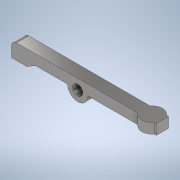
# Autodesk Inventor part: Peça8
Saved by Autodesk Inventor 2021 (Build 250183000, 183)
## iProperties
Created: 2021-07-18
Part Number: Peça8
Material: Liga de aço
Document SubType Name: Modeling
Designer: Giovanni
Density: 7.73 g/cm^3
Appearance: Galvanizado
Author: Giovanni
Autodesk Inventor part; units mm, degrees
ref_plane "YZ Plane" through (0, 0, 0) normal (1, 0, 0) x (0, 1, 0)
ref_plane "XZ Plane" through (0, 0, 0) normal (0, 1, 0) x (-1, 0, 0)
ref_plane "XY Plane" through (0, 0, 0) normal (0, 0, 1) x (1, 0, 0)
sketch "Esboço1" plane through (0, 0, 0) normal (0, 0, 1) x (1, 0, 0)
  arc A0 (-10, 0) -> (10, 0) centre (0, 0) ccw
  line L0 (10, 0) -> (77, 0)
  line L1 (77, 0) -> (77, 10)
  line L2 (77, 10) -> (-65, 10)
  line L3 (-65, 10) -> (-65, -5)
  line L4 (-65, -5) -> (-50, -5)
  line L5 (-50, -5) -> (-41.3397, 0)
  line L6 (-41.3397, 0) -> (-10, 0)
  dimension "d0" = 20
  dimension "d1" = 142
  dimension "d2" = 77
  dimension "d3" = 15
  dimension "d4" = 30
  dimension "d5" = 10
  dimension "d6" = 15
  constraints: 14 end point, 3 perpendicular, 2 horizontal, 2 horizontal alignment, 2 point on circle, 1 centre point, 1 coincident, 1 parallel
  measures "d0" diameter of A0
  measures "d1" distance of L1.end L2.end
  measures "d2" distance from line of L1 point (0, 0)
  measures "d3" distance of L3.end L4.end
  measures "d4" angle of L6 L5
  measures "d5" distance of L0.end L1.end
  measures "d6" distance of L2.end L3.end
extrude "Extrusão1" add sketch "Esboço1" along normal mid plane 12
fillet "Arredondamento1" radius 5 1 edges at (-65, 10, 0)
sketch "Esboço2" plane through (0, 0, 6) normal (0, 0, 1) x (1, 0, 0)
  circle A0 centre (0, 0) radius 5
  dimension "d10" = 10
  constraints: 1 centre point, 1 coincident
  measures "d10" diameter of A0
extrude "Extrusão2" cut sketch "Esboço2" against normal through all
sketch "Esboço3" plane through (77, 10, 6) normal (0, 1, 0) x (1, 0, 0)
  circle A0 centre (-10, 6) radius 10
  line L0 (0, 12) -> (0, 0) projected
  line L1 (-137, 0) -> (-137, 12) projected
  point P0 (-77, 6)
  point P1 (-137, 6)
  dimension "d13" = 20
  dimension "d14" = 10
  constraints: 1 centre point, 1 horizontal alignment, 1 midpoint
  measures "d13" diameter of A0
  measures "d14" distance from line of L0 A0.centre
extrude "Extrusão3" add sketch "Esboço3" against normal blind 10
